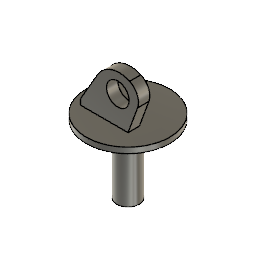
Assembly (Autodesk Fusion 360 archive; units mm, degrees)
design "Z rotation"
Autodesk Fusion 360 part; units mm, degrees
(part 1 of 5)
cylinder "CylinderPrimitive1" add diameter 20 height 60 placed x (1, 0, 0) y (0, 1, 0) z (0, 0, 1) at (0, 0, 0)
sketch "Sketch2" plane through (0, 0, 60) normal (0, 0, 1) x (-1, 0, 0)
  circle A0 centre (0, 0) radius 10
  circle A1 centre (0, 0) radius 37
  dimension "d3" = 74
  constraint coincident A0.centre A1.centre
  measures "d3" diameter of A1
extrude "Extrude1" add sketch "Sketch2" along normal blind 5 contours A0 | A1
sketch "Sketch3" plane through (0, 0, 0) normal (0, 1, 0) x (1, 0, 0)
  line L0 (-37, -65) -> (37, -65)
  line L1 (-27, -65) -> (-27, -70)
  line L2 (-27, -70) -> (-12, -95.9808)
  line L3 (-27, -70) -> (3, -70) construction
  line L4 (15.0513, -65) -> (23.4704, -88.1312)
  line L5 (-12, -95.9808) -> (26.3274, -95.9808) construction
  arc A0 (-12, -95.9808) -> (16.4497, -105.0022) centre (7.1637, -84.9166) ccw
  arc A1 (16.4497, -105.0022) -> (23.4704, -88.1312) centre (10.7845, -92.7484) ccw
  dimension "d6" = 5
  dimension "d8" = 30
  dimension "d9" = 10
  dimension "d12" = 74
  dimension "d15" = 60
  dimension "d16" = 70
  dimension "d17" = 13.5
  constraint coincident L0 L1.start
  constraint perpendicular L0 L1
  constraint horizontal L3
  constraint coincident L0 L4.start
  constraint horizontal L5
  constraint tangent L2 A0
  constraint coincident L4 L5.end
  constraint coincident L5.end A0
  constraint tangent L4 A1
  constraint tangent A0 A1
  measures "d6" distance of L1.start L1.end
  measures "d8" distance of L1.end L2.end
  measures "d9" distance of L0.start L1.start
  measures "d12" distance of L0.start L0.end
  measures "d15" angle of L2 L3
  measures "d16" angle of L0 L4
  measures "d17" radius of A1
extrude "Extrude2" add sketch "Sketch3" against normal blind 10 from surface at -5
hole "Hole1" at (6, -15, 90) direction (0, 1, 0) diameter 20 end through all

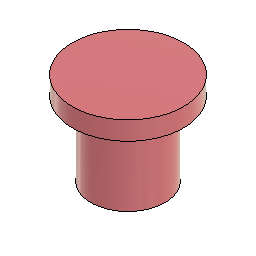
design "Pin"
Autodesk Fusion 360 part; units mm, degrees
sketch "Sketch1" plane through (0, 0, 0) normal (0, 0, 1) x (1, 0, 0)
  circle A0 centre (0, 0) radius 10
  dimension "d1" = 20
  constraint coincident A0.centre origin
  measures "d1" diameter of A0
extrude "Extrude1" add sketch "Sketch1" along normal blind 20
sketch "Sketch2" plane through (0, 0, 20) normal (0, 0, 1) x (-1, 0, 0)
  circle A0 centre (0, 0) radius 10
  circle A1 centre (0, 0) radius 15
  dimension "d4" = 30
  constraint coincident A0.centre A1.centre
  measures "d4" diameter of A1
extrude "Extrude2" add sketch "Sketch2" along normal blind 5 contours A0 | A1

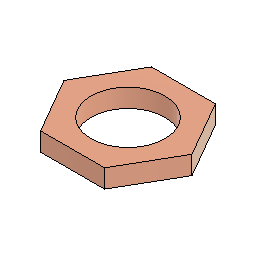
design "Hex"
Autodesk Fusion 360 part; units mm, degrees
sketch "Sketch1" plane through (0, 0, 0) normal (0, 0, 1) x (1, 0, 0)
  line L0 (8.6603, -15) -> (17.3205, 0)
  line L1 (17.3205, 0) -> (8.6603, 15)
  line L2 (8.6603, 15) -> (-8.6603, 15)
  line L3 (-8.6603, 15) -> (-17.3205, 0)
  line L4 (-17.3205, 0) -> (-8.6603, -15)
  line L5 (-8.6603, -15) -> (8.6603, -15)
  dimension "d1" = 15
  measures "d1" distance of origin L5
extrude "Extrude1" add sketch "Sketch1" along normal blind 5
hole "Hole1" at (0, 0, 5) direction (0, 0, -1) diameter 20 depth 20 tip angle 118

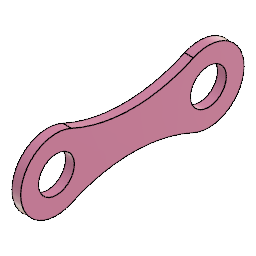
design "Yoke"
Autodesk Fusion 360 part; units mm, degrees
sketch "Sketch1" plane through (0, 0, 0) normal (1, 0, 0) x (0, 1, 0)
  circle A0 centre (0, 0) radius 20
  circle A1 centre (0, 0) radius 10
  line L0 (0, 0) -> (85, 0) construction
  circle A2 centre (85, 0) radius 20
  circle A3 centre (85, 0) radius 10
  arc A4 (8.3775, 18.1609) -> (76.6225, 18.1609) centre (42.5, 92.1318) ccw
  arc A5 (76.6225, -18.1609) -> (8.3775, -18.1609) centre (42.5, -92.1318) ccw
  dimension "d1" = 40
  dimension "d2" = 20
  dimension "d3" = 85
  dimension "d4" = 40
  dimension "d5" = 20
  constraint coincident A0.centre A1.centre
  constraint concentric A0 A1
  constraint horizontal L0
  constraint coincident L0.end A2.centre
  constraint concentric A2 A3
  constraint tangent A0 A4
  constraint tangent A2 A4
  constraint symmetric L0 A4 A5
  constraint coincident A2 A4.end
  constraint coincident A0 A4.start
  constraint coincident A0 A5.end
  constraint coincident A2 A5.start
  measures "d1" diameter of A0
  measures "d2" diameter of A1
  measures "d3" distance of A0.centre L0.end
  measures "d4" diameter of A2
  measures "d5" diameter of A3
extrude "Extrude1" add sketch "Sketch1" along normal blind 5

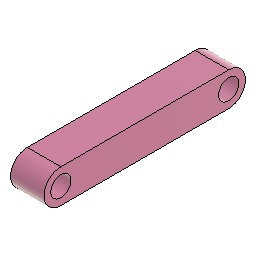
design "SmallYoke"
Autodesk Fusion 360 part; units mm, degrees
sketch "Sketch1" plane through (0, 0, 0) normal (1, 0, 0) x (0, 1, 0)
  circle A0 centre (0, 0) radius 2.5
  circle A1 centre (0, 0) radius 1.5
  line L0 (0, 0) -> (25, 0) construction
  circle A2 centre (25, 0) radius 2.5
  circle A3 centre (25, 0) radius 1.5
  line L1 (0, 2.5) -> (25, 2.5)
  line L2 (0, -2.5) -> (25, -2.5)
  dimension "d1" = 5
  dimension "d2" = 3
  dimension "d3" = 25
  dimension "d4" = 5
  dimension "d5" = 3
  constraint coincident A0.centre A1.centre
  constraint concentric A0 A1
  constraint horizontal L0
  constraint coincident L0.end A2.centre
  constraint concentric A2 A3
  constraint tangent A0 L1
  constraint tangent A2 L1
  constraint coincident A0 L1.start
  constraint coincident A2 L1.end
  constraint symmetric L0 L1.start L2.start
  constraint symmetric L0 L1.end L2.end
  measures "d1" diameter of A0
  measures "d2" diameter of A1
  measures "d3" distance of A0.centre L0.end
  measures "d4" diameter of A2
  measures "d5" diameter of A3
extrude "Extrude1" add sketch "Sketch1" along normal blind 5

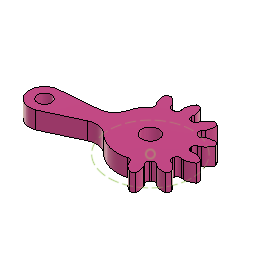
design "Spur Gear-Left"
description: Spur Gear; Module: 2.0; Num Teeth: 12; Pressure Angle: 20.0; Backlash: 0.00 mm
Autodesk Fusion 360 part; units mm, degrees
derive "DerivedContext1" from "Assembly v8"
sketch "Sketch1" plane through (0, 0, 0) normal (0, 0, 1) x (1, 0, 0) in component "Spur Gear (12 teeth)"
  circle A0 centre (0, 0) radius 9.5492
  circle A1 centre (0, 0) radius 2.5
extrude "Extrude1" add sketch "Sketch1" along normal blind 5 in component "Spur Gear (12 teeth)"
sketch "Sketch2" plane through (0, 0, 0) normal (0, 0, 1) x (1, 0, 0) in component "Spur Gear (12 teeth)"
  spline S0 degree 5 poles (11.1567, -1.6383) (11.1647, -1.6395) (11.1807, -1.6416) (11.2048, -1.6439) (11.237, -1.6456) (11.2774, -1.6458) (11.318, -1.6445) (11.3587, -1.6423) (11.3994, -1.6396) (11.4401, -1.6366) (11.4809, -1.6333) (11.5218, -1.6295) (11.5626, -1.625) (11.6035, -1.6199) (11.6445, -1.614) (11.6854, -1.6075) (11.7264, -1.6005) (11.7674, -1.5929) (11.8084, -1.585) (11.8494, -1.5766) (11.8905, -1.5678) (11.9315, -1.5587) (11.9725, -1.5491) (12.0135, -1.539) (12.0545, -1.5285) (12.0956, -1.5175) (12.1366, -1.5062) (12.1776, -1.4944) (12.2186, -1.4823) (12.2595, -1.4698) (12.3005, -1.4569) (12.3414, -1.4437) (12.3824, -1.4301) (12.4233, -1.4161) (12.4641, -1.4018) (12.505, -1.3871) (12.5458, -1.372) (12.5866, -1.3566) (12.6274, -1.3409) (12.6681, -1.3248) (12.7088, -1.3084) (12.7495, -1.2917) (12.7902, -1.2746) (12.8308, -1.2572) (12.8713, -1.2395) (12.9119, -1.2215) (12.9523, -1.2031) (12.9928, -1.1844) (13.0332, -1.1654) (13.0735, -1.1461) (13.1138, -1.1265) (13.1541, -1.1066) (13.1943, -1.0863) (13.2345, -1.0658) (13.2746, -1.045) (13.3146, -1.0239) (13.3546, -1.0024) (13.3946, -0.9807) (13.4344, -0.9587) (13.4743, -0.9364) (13.514, -0.9138) (13.5538, -0.8909) (13.5934, -0.8678) (13.633, -0.8443) (13.6725, -0.8206) (13.712, -0.7966) (13.7514, -0.7723) (13.7907, -0.7477) (13.8299, -0.7229) (13.8691, -0.6978) (13.9082, -0.6724) (13.9395, -0.6518) (13.9629, -0.6363) (13.9784, -0.6259) (13.9862, -0.6207) knots 0 0 0 0 0 0 0.01428571 0.02857143 0.04285714 0.05714286 0.07142857 0.08571429 0.1 0.11428571 0.12857143 0.14285714 0.15714286 0.17142857 0.18571429 0.2 0.21428571 0.22857143 0.24285714 0.25714286 0.27142857 0.28571429 0.3 0.31428571 0.32857143 0.34285714 0.35714286 0.37142857 0.38571429 0.4 0.41428571 0.42857143 0.44285714 0.45714286 0.47142857 0.48571429 0.5 0.51428571 0.52857143 0.54285714 0.55714286 0.57142857 0.58571429 0.6 0.61428571 0.62857143 0.64285714 0.65714286 0.67142857 0.68571429 0.7 0.71428571 0.72857143 0.74285714 0.75714286 0.77142857 0.78571429 0.8 0.81428571 0.82857143 0.84285714 0.85714286 0.87142857 0.88571429 0.9 0.91428571 0.92857143 0.94285714 0.95714286 0.97142857 0.98571429 1 1 1 1 1 1
  spline S1 degree 5 poles (11.1567, 1.6383) (11.1647, 1.6395) (11.1807, 1.6416) (11.2048, 1.6439) (11.237, 1.6456) (11.2774, 1.6458) (11.318, 1.6445) (11.3587, 1.6423) (11.3994, 1.6396) (11.4401, 1.6366) (11.4809, 1.6333) (11.5218, 1.6295) (11.5626, 1.625) (11.6035, 1.6199) (11.6445, 1.614) (11.6854, 1.6075) (11.7264, 1.6005) (11.7674, 1.5929) (11.8084, 1.585) (11.8494, 1.5766) (11.8905, 1.5678) (11.9315, 1.5587) (11.9725, 1.5491) (12.0135, 1.539) (12.0545, 1.5285) (12.0956, 1.5175) (12.1366, 1.5062) (12.1776, 1.4944) (12.2186, 1.4823) (12.2595, 1.4698) (12.3005, 1.4569) (12.3414, 1.4437) (12.3824, 1.4301) (12.4233, 1.4161) (12.4641, 1.4018) (12.505, 1.3871) (12.5458, 1.372) (12.5866, 1.3566) (12.6274, 1.3409) (12.6681, 1.3248) (12.7088, 1.3084) (12.7495, 1.2917) (12.7902, 1.2746) (12.8308, 1.2572) (12.8713, 1.2395) (12.9119, 1.2215) (12.9523, 1.2031) (12.9928, 1.1844) (13.0332, 1.1654) (13.0735, 1.1461) (13.1138, 1.1265) (13.1541, 1.1066) (13.1943, 1.0863) (13.2345, 1.0658) (13.2746, 1.045) (13.3146, 1.0239) (13.3546, 1.0024) (13.3946, 0.9807) (13.4344, 0.9587) (13.4743, 0.9364) (13.514, 0.9138) (13.5538, 0.8909) (13.5934, 0.8678) (13.633, 0.8443) (13.6725, 0.8206) (13.712, 0.7966) (13.7514, 0.7723) (13.7907, 0.7477) (13.8299, 0.7229) (13.8691, 0.6978) (13.9082, 0.6724) (13.9395, 0.6518) (13.9629, 0.6363) (13.9784, 0.6259) (13.9862, 0.6207) knots 0 0 0 0 0 0 0.01428571 0.02857143 0.04285714 0.05714286 0.07142857 0.08571429 0.1 0.11428571 0.12857143 0.14285714 0.15714286 0.17142857 0.18571429 0.2 0.21428571 0.22857143 0.24285714 0.25714286 0.27142857 0.28571429 0.3 0.31428571 0.32857143 0.34285714 0.35714286 0.37142857 0.38571429 0.4 0.41428571 0.42857143 0.44285714 0.45714286 0.47142857 0.48571429 0.5 0.51428571 0.52857143 0.54285714 0.55714286 0.57142857 0.58571429 0.6 0.61428571 0.62857143 0.64285714 0.65714286 0.67142857 0.68571429 0.7 0.71428571 0.72857143 0.74285714 0.75714286 0.77142857 0.78571429 0.8 0.81428571 0.82857143 0.84285714 0.85714286 0.87142857 0.88571429 0.9 0.91428571 0.92857143 0.94285714 0.95714286 0.97142857 0.98571429 1 1 1 1 1 1
  arc A0 (13.9862, -0.6207) -> (13.9862, 0.6207) centre (0, 0) ccw
  line L0 (9.438, -1.3874) -> (11.1567, -1.6383)
  line L1 (9.438, 1.3874) -> (11.1567, 1.6383)
  line L2 (9.438, -1.3874) -> (9.438, 1.3874)
  point P0 (11.3527, -1.6425)
  point P1 (11.5515, -1.6261)
  point P2 (11.7521, -1.5957)
  point P3 (11.954, -1.5533)
  point P4 (12.1568, -1.5003)
  point P5 (12.3603, -1.4374)
  point P6 (12.5642, -1.3651)
  point P7 (12.7683, -1.2838)
  point P8 (12.9724, -1.1938)
  point P9 (13.1764, -1.0953)
  point P10 (13.3799, -0.9887)
  point P11 (13.5828, -0.8739)
  point P12 (13.785, -0.7512)
  point P13 (11.3527, 1.6425)
  point P14 (11.5515, 1.6261)
  point P15 (11.7521, 1.5957)
  point P16 (11.954, 1.5533)
  point P17 (12.1568, 1.5003)
  point P18 (12.3603, 1.4374)
  point P19 (12.5642, 1.3651)
  point P20 (12.7683, 1.2838)
  point P21 (12.9724, 1.1938)
  point P22 (13.1764, 1.0953)
  point P23 (13.3799, 0.9887)
  point P24 (13.5828, 0.8739)
  point P25 (13.785, 0.7512)
extrude "Extrude2" add sketch "Sketch2" along normal blind 5 in component "Spur Gear (12 teeth)"
fillet "Fillet1" radius 1 2 edges at (9.4477, -1.3888, 2.5) (9.4477, 1.3888, 2.5) in component "Spur Gear (12 teeth)"
pattern_circular "C-Pattern1" count 12 over 360 about axis through (0, 0, 0) along (0, 0, 1) of "Extrude2", "Fillet1" in component "Spur Gear (12 teeth)"
sketch "Sketch3" plane through (0, 0, 0) normal (0, 0, 1) x (1, 0, 0) in component "Spur Gear (12 teeth)"
  circle A0 centre (0, 0) radius 12 construction
sketch "Sketch1 (2)" plane through (0, 0, 5) normal (0, 0, 1) x (-1, 0, 0)
  arc A0 (-9.1699, 2.6646) -> (-9.2737, 2.2773) centre (0, 0) ccw
  arc A1 (-10.3893, 1.5263) -> (-9.2737, 2.2773) centre (-10.2448, 2.5158) ccw
  line L0 (-10.3893, 1.5263) -> (-11.1567, 1.6383)
  spline S0 degree 5 poles (-11.1567, 1.6383) (-11.1647, 1.6395) (-11.1807, 1.6416) (-11.2048, 1.6439) (-11.237, 1.6456) (-11.2774, 1.6458) (-11.318, 1.6445) (-11.3587, 1.6423) (-11.3994, 1.6396) (-11.4401, 1.6366) (-11.4809, 1.6333) (-11.5218, 1.6295) (-11.5626, 1.625) (-11.6035, 1.6199) (-11.6445, 1.614) (-11.6854, 1.6075) (-11.7264, 1.6005) (-11.7674, 1.5929) (-11.8084, 1.585) (-11.8494, 1.5766) (-11.8905, 1.5678) (-11.9315, 1.5587) (-11.9725, 1.5491) (-12.0135, 1.539) (-12.0545, 1.5285) (-12.0956, 1.5175) (-12.1366, 1.5062) (-12.1776, 1.4944) (-12.2186, 1.4823) (-12.2595, 1.4698) (-12.3005, 1.4569) (-12.3414, 1.4437) (-12.3824, 1.4301) (-12.4233, 1.4161) (-12.4641, 1.4018) (-12.505, 1.3871) (-12.5458, 1.372) (-12.5866, 1.3566) (-12.6274, 1.3409) (-12.6681, 1.3248) (-12.7088, 1.3084) (-12.7495, 1.2917) (-12.7902, 1.2746) (-12.8308, 1.2572) (-12.8713, 1.2395) (-12.9119, 1.2215) (-12.9523, 1.2031) (-12.9928, 1.1844) (-13.0332, 1.1654) (-13.0735, 1.1461) (-13.1138, 1.1265) (-13.1541, 1.1066) (-13.1943, 1.0863) (-13.2345, 1.0658) (-13.2746, 1.045) (-13.3146, 1.0239) (-13.3546, 1.0024) (-13.3946, 0.9807) (-13.4344, 0.9587) (-13.4743, 0.9364) (-13.514, 0.9138) (-13.5538, 0.8909) (-13.5934, 0.8678) (-13.633, 0.8443) (-13.6725, 0.8206) (-13.712, 0.7966) (-13.7514, 0.7723) (-13.7907, 0.7477) (-13.8299, 0.7229) (-13.8691, 0.6978) (-13.9082, 0.6724) (-13.9395, 0.6518) (-13.9629, 0.6363) (-13.9784, 0.6259) (-13.9862, 0.6207) knots 0 0 0 0 0 0 0.01428571 0.02857143 0.04285714 0.05714286 0.07142857 0.08571429 0.1 0.11428571 0.12857143 0.14285714 0.15714286 0.17142857 0.18571429 0.2 0.21428571 0.22857143 0.24285714 0.25714286 0.27142857 0.28571429 0.3 0.31428571 0.32857143 0.34285714 0.35714286 0.37142857 0.38571429 0.4 0.41428571 0.42857143 0.44285714 0.45714286 0.47142857 0.48571429 0.5 0.51428571 0.52857143 0.54285714 0.55714286 0.57142857 0.58571429 0.6 0.61428571 0.62857143 0.64285714 0.65714286 0.67142857 0.68571429 0.7 0.71428571 0.72857143 0.74285714 0.75714286 0.77142857 0.78571429 0.8 0.81428571 0.82857143 0.84285714 0.85714286 0.87142857 0.88571429 0.9 0.91428571 0.92857143 0.94285714 0.95714286 0.97142857 0.98571429 1 1 1 1 1 1
  arc A2 (-13.9862, 0.6207) -> (-13.9862, -0.6207) centre (0, 0) ccw
  spline S1 degree 5 poles (-13.9862, -0.6207) (-13.9784, -0.6259) (-13.9629, -0.6363) (-13.9395, -0.6518) (-13.9082, -0.6724) (-13.8691, -0.6978) (-13.8299, -0.7229) (-13.7907, -0.7477) (-13.7514, -0.7723) (-13.712, -0.7966) (-13.6725, -0.8206) (-13.633, -0.8443) (-13.5934, -0.8678) (-13.5538, -0.8909) (-13.514, -0.9138) (-13.4743, -0.9364) (-13.4344, -0.9587) (-13.3946, -0.9807) (-13.3546, -1.0024) (-13.3146, -1.0239) (-13.2746, -1.045) (-13.2345, -1.0658) (-13.1943, -1.0863) (-13.1541, -1.1066) (-13.1138, -1.1265) (-13.0735, -1.1461) (-13.0332, -1.1654) (-12.9928, -1.1844) (-12.9523, -1.2031) (-12.9119, -1.2215) (-12.8713, -1.2395) (-12.8308, -1.2572) (-12.7902, -1.2746) (-12.7495, -1.2917) (-12.7088, -1.3084) (-12.6681, -1.3248) (-12.6274, -1.3409) (-12.5866, -1.3566) (-12.5458, -1.372) (-12.505, -1.3871) (-12.4641, -1.4018) (-12.4233, -1.4161) (-12.3824, -1.4301) (-12.3414, -1.4437) (-12.3005, -1.4569) (-12.2595, -1.4698) (-12.2186, -1.4823) (-12.1776, -1.4944) (-12.1366, -1.5062) (-12.0956, -1.5175) (-12.0545, -1.5285) (-12.0135, -1.539) (-11.9725, -1.5491) (-11.9315, -1.5587) (-11.8905, -1.5678) (-11.8494, -1.5766) (-11.8084, -1.585) (-11.7674, -1.5929) (-11.7264, -1.6005) (-11.6854, -1.6075) (-11.6445, -1.614) (-11.6035, -1.6199) (-11.5626, -1.625) (-11.5218, -1.6295) (-11.4809, -1.6333) (-11.4401, -1.6366) (-11.3994, -1.6396) (-11.3587, -1.6423) (-11.318, -1.6445) (-11.2774, -1.6458) (-11.237, -1.6456) (-11.2048, -1.6439) (-11.1807, -1.6416) (-11.1647, -1.6395) (-11.1567, -1.6383) knots -1 -1 -1 -1 -1 -1 -0.98571429 -0.97142857 -0.95714286 -0.94285714 -0.92857143 -0.91428571 -0.9 -0.88571429 -0.87142857 -0.85714286 -0.84285714 -0.82857143 -0.81428571 -0.8 -0.78571429 -0.77142857 -0.75714286 -0.74285714 -0.72857143 -0.71428571 -0.7 -0.68571429 -0.67142857 -0.65714286 -0.64285714 -0.62857143 -0.61428571 -0.6 -0.58571429 -0.57142857 -0.55714286 -0.54285714 -0.52857143 -0.51428571 -0.5 -0.48571429 -0.47142857 -0.45714286 -0.44285714 -0.42857143 -0.41428571 -0.4 -0.38571429 -0.37142857 -0.35714286 -0.34285714 -0.32857143 -0.31428571 -0.3 -0.28571429 -0.27142857 -0.25714286 -0.24285714 -0.22857143 -0.21428571 -0.2 -0.18571429 -0.17142857 -0.15714286 -0.14285714 -0.12857143 -0.11428571 -0.1 -0.08571429 -0.07142857 -0.05714286 -0.04285714 -0.02857143 -0.01428571 0 0 0 0 0 0
  line L1 (-11.1567, -1.6383) -> (-10.3893, -1.5263)
  arc A3 (-9.2737, -2.2773) -> (-10.3893, -1.5263) centre (-10.2448, -2.5158) ccw
  arc A4 (-9.2737, -2.2773) -> (-9.1699, -2.6646) centre (0, 0) ccw
  arc A5 (-9.7605, -3.8729) -> (-9.1699, -2.6646) centre (-10.1302, -2.9437) ccw
  line L2 (-9.7605, -3.8729) -> (-10.4811, -4.1595)
  spline S2 degree 5 poles (-10.4811, -4.1595) (-10.4886, -4.1625) (-10.5035, -4.1687) (-10.5256, -4.1787) (-10.5543, -4.1933) (-10.5894, -4.2134) (-10.6239, -4.2349) (-10.658, -4.2571) (-10.692, -4.2797) (-10.7258, -4.3027) (-10.7594, -4.326) (-10.7929, -4.3497) (-10.826, -4.374) (-10.8589, -4.3989) (-10.8914, -4.4244) (-10.9236, -4.4505) (-10.9556, -4.4772) (-10.9873, -4.5042) (-11.0189, -4.5316) (-11.0502, -4.5593) (-11.0814, -4.5874) (-11.1123, -4.6159) (-11.143, -4.6447) (-11.1735, -4.674) (-11.2038, -4.7036) (-11.2338, -4.7336) (-11.2637, -4.7639) (-11.2933, -4.7946) (-11.3227, -4.8256) (-11.352, -4.8569) (-11.381, -4.8885) (-11.4099, -4.9204) (-11.4385, -4.9527) (-11.4669, -4.9852) (-11.4952, -5.0181) (-11.5232, -5.0512) (-11.551, -5.0847) (-11.5787, -5.1184) (-11.6061, -5.1524) (-11.6334, -5.1867) (-11.6604, -5.2213) (-11.6873, -5.2561) (-11.7139, -5.2912) (-11.7404, -5.3266) (-11.7666, -5.3622) (-11.7927, -5.3981) (-11.8186, -5.4343) (-11.8443, -5.4707) (-11.8698, -5.5073) (-11.8951, -5.5442) (-11.9202, -5.5813) (-11.9451, -5.6187) (-11.9698, -5.6563) (-11.9943, -5.6942) (-12.0186, -5.7323) (-12.0427, -5.7706) (-12.0667, -5.8092) (-12.0904, -5.848) (-12.1139, -5.887) (-12.1373, -5.9262) (-12.1604, -5.9656) (-12.1834, -6.0053) (-12.2061, -6.0452) (-12.2287, -6.0853) (-12.251, -6.1256) (-12.2732, -6.1661) (-12.2952, -6.2069) (-12.3169, -6.2478) (-12.3385, -6.2889) (-12.3599, -6.3303) (-12.3811, -6.3718) (-12.3979, -6.4052) (-12.4104, -6.4304) (-12.4186, -6.4472) (-12.4228, -6.4556) knots 0 0 0 0 0 0 0.01428571 0.02857143 0.04285714 0.05714286 0.07142857 0.08571429 0.1 0.11428571 0.12857143 0.14285714 0.15714286 0.17142857 0.18571429 0.2 0.21428571 0.22857143 0.24285714 0.25714286 0.27142857 0.28571429 0.3 0.31428571 0.32857143 0.34285714 0.35714286 0.37142857 0.38571429 0.4 0.41428571 0.42857143 0.44285714 0.45714286 0.47142857 0.48571429 0.5 0.51428571 0.52857143 0.54285714 0.55714286 0.57142857 0.58571429 0.6 0.61428571 0.62857143 0.64285714 0.65714286 0.67142857 0.68571429 0.7 0.71428571 0.72857143 0.74285714 0.75714286 0.77142857 0.78571429 0.8 0.81428571 0.82857143 0.84285714 0.85714286 0.87142857 0.88571429 0.9 0.91428571 0.92857143 0.94285714 0.95714286 0.97142857 0.98571429 1 1 1 1 1 1
  arc A6 (-12.4228, -6.4556) -> (-11.8021, -7.5307) centre (0, 0) ccw
  spline S3 degree 5 poles (-11.8021, -7.5307) (-11.7927, -7.5313) (-11.774, -7.5325) (-11.746, -7.5342) (-11.7087, -7.5364) (-11.6621, -7.5388) (-11.6156, -7.541) (-11.5692, -7.5429) (-11.5229, -7.5445) (-11.4766, -7.5458) (-11.4305, -7.5469) (-11.3844, -7.5477) (-11.3384, -7.5482) (-11.2924, -7.5484) (-11.2466, -7.5484) (-11.2009, -7.5481) (-11.1552, -7.5475) (-11.1097, -7.5466) (-11.0642, -7.5454) (-11.0189, -7.544) (-10.9736, -7.5423) (-10.9285, -7.5403) (-10.8834, -7.538) (-10.8385, -7.5354) (-10.7937, -7.5325) (-10.7489, -7.5293) (-10.7044, -7.5259) (-10.6599, -7.5221) (-10.6155, -7.5181) (-10.5713, -7.5137) (-10.5271, -7.5091) (-10.4832, -7.5042) (-10.4393, -7.4989) (-10.3956, -7.4934) (-10.352, -7.4876) (-10.3085, -7.4814) (-10.2652, -7.475) (-10.222, -7.4682) (-10.179, -7.4611) (-10.1361, -7.4538) (-10.0934, -7.4461) (-10.0508, -7.438) (-10.0084, -7.4297) (-9.9662, -7.421) (-9.9241, -7.412) (-9.8822, -7.4027) (-9.8404, -7.393) (-9.7989, -7.383) (-9.7575, -7.3727) (-9.7163, -7.362) (-9.6753, -7.351) (-9.6345, -7.3396) (-9.594, -7.3278) (-9.5536, -7.3156) (-9.5135, -7.303) (-9.4736, -7.2901) (-9.4339, -7.2768) (-9.3944, -7.2632) (-9.3551, -7.2492) (-9.3161, -7.2349) (-9.2774, -7.22) (-9.239, -7.2046) (-9.201, -7.1886) (-9.1634, -7.172) (-9.1261, -7.1549) (-9.0891, -7.1374) (-9.0523, -7.1196) (-9.0157, -7.1016) (-8.9794, -7.0831) (-8.9437, -7.064) (-8.9087, -7.0436) (-8.8816, -7.0261) (-8.862, -7.012) (-8.8491, -7.0022) (-8.8428, -6.9972) knots -1 -1 -1 -1 -1 -1 -0.98571429 -0.97142857 -0.95714286 -0.94285714 -0.92857143 -0.91428571 -0.9 -0.88571429 -0.87142857 -0.85714286 -0.84285714 -0.82857143 -0.81428571 -0.8 -0.78571429 -0.77142857 -0.75714286 -0.74285714 -0.72857143 -0.71428571 -0.7 -0.68571429 -0.67142857 -0.65714286 -0.64285714 -0.62857143 -0.61428571 -0.6 -0.58571429 -0.57142857 -0.55714286 -0.54285714 -0.52857143 -0.51428571 -0.5 -0.48571429 -0.47142857 -0.45714286 -0.44285714 -0.42857143 -0.41428571 -0.4 -0.38571429 -0.37142857 -0.35714286 -0.34285714 -0.32857143 -0.31428571 -0.3 -0.28571429 -0.27142857 -0.25714286 -0.24285714 -0.22857143 -0.21428571 -0.2 -0.18571429 -0.17142857 -0.15714286 -0.14285714 -0.12857143 -0.11428571 -0.1 -0.08571429 -0.07142857 -0.05714286 -0.04285714 -0.02857143 -0.01428571 0 0 0 0 0 0
  line L3 (-8.8428, -6.9972) -> (-8.2343, -6.5164)
  arc A7 (-6.8926, -6.609) -> (-8.2343, -6.5164) centre (-7.6144, -7.3011) ccw
  arc A8 (-6.8926, -6.609) -> (-6.609, -6.8926) centre (0, 0) ccw
  arc A9 (-6.5164, -8.2343) -> (-6.609, -6.8926) centre (-7.3011, -7.6144) ccw
  line L4 (-6.5164, -8.2343) -> (-6.9972, -8.8428)
  spline S4 degree 5 poles (-6.9972, -8.8428) (-7.0022, -8.8491) (-7.012, -8.862) (-7.0261, -8.8816) (-7.0436, -8.9087) (-7.064, -8.9437) (-7.0831, -8.9794) (-7.1016, -9.0157) (-7.1196, -9.0523) (-7.1374, -9.0891) (-7.1549, -9.1261) (-7.172, -9.1634) (-7.1886, -9.201) (-7.2046, -9.239) (-7.22, -9.2774) (-7.2349, -9.3161) (-7.2492, -9.3551) (-7.2632, -9.3944) (-7.2768, -9.4339) (-7.2901, -9.4736) (-7.303, -9.5135) (-7.3156, -9.5536) (-7.3278, -9.594) (-7.3396, -9.6345) (-7.351, -9.6753) (-7.362, -9.7163) (-7.3727, -9.7575) (-7.383, -9.7989) (-7.393, -9.8404) (-7.4027, -9.8822) (-7.412, -9.9241) (-7.421, -9.9662) (-7.4297, -10.0084) (-7.438, -10.0508) (-7.4461, -10.0934) (-7.4538, -10.1361) (-7.4611, -10.179) (-7.4682, -10.222) (-7.475, -10.2652) (-7.4814, -10.3085) (-7.4876, -10.352) (-7.4934, -10.3956) (-7.4989, -10.4393) (-7.5042, -10.4832) (-7.5091, -10.5271) (-7.5137, -10.5713) (-7.5181, -10.6155) (-7.5221, -10.6599) (-7.5259, -10.7044) (-7.5293, -10.7489) (-7.5325, -10.7937) (-7.5354, -10.8385) (-7.538, -10.8834) (-7.5403, -10.9285) (-7.5423, -10.9736) (-7.544, -11.0189) (-7.5454, -11.0642) (-7.5466, -11.1097) (-7.5475, -11.1552) (-7.5481, -11.2009) (-7.5484, -11.2466) (-7.5484, -11.2924) (-7.5482, -11.3384) (-7.5477, -11.3844) (-7.5469, -11.4305) (-7.5458, -11.4766) (-7.5445, -11.5229) (-7.5429, -11.5692) (-7.541, -11.6156) (-7.5388, -11.6621) (-7.5364, -11.7087) (-7.5342, -11.746) (-7.5325, -11.774) (-7.5313, -11.7927) (-7.5307, -11.8021) knots 0 0 0 0 0 0 0.01428571 0.02857143 0.04285714 0.05714286 0.07142857 0.08571429 0.1 0.11428571 0.12857143 0.14285714 0.15714286 0.17142857 0.18571429 0.2 0.21428571 0.22857143 0.24285714 0.25714286 0.27142857 0.28571429 0.3 0.31428571 0.32857143 0.34285714 0.35714286 0.37142857 0.38571429 0.4 0.41428571 0.42857143 0.44285714 0.45714286 0.47142857 0.48571429 0.5 0.51428571 0.52857143 0.54285714 0.55714286 0.57142857 0.58571429 0.6 0.61428571 0.62857143 0.64285714 0.65714286 0.67142857 0.68571429 0.7 0.71428571 0.72857143 0.74285714 0.75714286 0.77142857 0.78571429 0.8 0.81428571 0.82857143 0.84285714 0.85714286 0.87142857 0.88571429 0.9 0.91428571 0.92857143 0.94285714 0.95714286 0.97142857 0.98571429 1 1 1 1 1 1
  arc A10 (-7.5307, -11.8021) -> (-6.4556, -12.4228) centre (0, 0) ccw
  spline S5 degree 5 poles (-6.4556, -12.4228) (-6.4472, -12.4186) (-6.4304, -12.4104) (-6.4052, -12.3979) (-6.3718, -12.3811) (-6.3303, -12.3599) (-6.2889, -12.3385) (-6.2478, -12.3169) (-6.2069, -12.2952) (-6.1661, -12.2732) (-6.1256, -12.251) (-6.0853, -12.2287) (-6.0452, -12.2061) (-6.0053, -12.1834) (-5.9656, -12.1604) (-5.9262, -12.1373) (-5.887, -12.1139) (-5.848, -12.0904) (-5.8092, -12.0667) (-5.7706, -12.0427) (-5.7323, -12.0186) (-5.6942, -11.9943) (-5.6563, -11.9698) (-5.6187, -11.9451) (-5.5813, -11.9202) (-5.5442, -11.8951) (-5.5073, -11.8698) (-5.4707, -11.8443) (-5.4343, -11.8186) (-5.3981, -11.7927) (-5.3622, -11.7666) (-5.3266, -11.7404) (-5.2912, -11.7139) (-5.2561, -11.6873) (-5.2213, -11.6604) (-5.1867, -11.6334) (-5.1524, -11.6061) (-5.1184, -11.5787) (-5.0847, -11.551) (-5.0512, -11.5232) (-5.0181, -11.4952) (-4.9852, -11.4669) (-4.9527, -11.4385) (-4.9204, -11.4099) (-4.8885, -11.381) (-4.8569, -11.352) (-4.8256, -11.3227) (-4.7946, -11.2933) (-4.7639, -11.2637) (-4.7336, -11.2338) (-4.7036, -11.2038) (-4.674, -11.1735) (-4.6447, -11.143) (-4.6159, -11.1123) (-4.5874, -11.0814) (-4.5593, -11.0502) (-4.5316, -11.0189) (-4.5042, -10.9873) (-4.4772, -10.9556) (-4.4505, -10.9236) (-4.4244, -10.8914) (-4.3989, -10.8589) (-4.374, -10.826) (-4.3497, -10.7929) (-4.326, -10.7594) (-4.3027, -10.7258) (-4.2797, -10.692) (-4.2571, -10.658) (-4.2349, -10.6239) (-4.2134, -10.5894) (-4.1933, -10.5543) (-4.1787, -10.5256) (-4.1687, -10.5035) (-4.1625, -10.4886) (-4.1595, -10.4811) knots -1 -1 -1 -1 -1 -1 -0.98571429 -0.97142857 -0.95714286 -0.94285714 -0.92857143 -0.91428571 -0.9 -0.88571429 -0.87142857 -0.85714286 -0.84285714 -0.82857143 -0.81428571 -0.8 -0.78571429 -0.77142857 -0.75714286 -0.74285714 -0.72857143 -0.71428571 -0.7 -0.68571429 -0.67142857 -0.65714286 -0.64285714 -0.62857143 -0.61428571 -0.6 -0.58571429 -0.57142857 -0.55714286 -0.54285714 -0.52857143 -0.51428571 -0.5 -0.48571429 -0.47142857 -0.45714286 -0.44285714 -0.42857143 -0.41428571 -0.4 -0.38571429 -0.37142857 -0.35714286 -0.34285714 -0.32857143 -0.31428571 -0.3 -0.28571429 -0.27142857 -0.25714286 -0.24285714 -0.22857143 -0.21428571 -0.2 -0.18571429 -0.17142857 -0.15714286 -0.14285714 -0.12857143 -0.11428571 -0.1 -0.08571429 -0.07142857 -0.05714286 -0.04285714 -0.02857143 -0.01428571 0 0 0 0 0 0
  line L5 (-4.1595, -10.4811) -> (-3.8729, -9.7605)
  arc A11 (-2.6646, -9.1699) -> (-3.8729, -9.7605) centre (-2.9437, -10.1302) ccw
  arc A12 (-2.6646, -9.1699) -> (-2.2773, -9.2737) centre (0, 0) ccw
  arc A13 (-1.5263, -10.3893) -> (-2.2773, -9.2737) centre (-2.5158, -10.2448) ccw
  line L6 (-1.5263, -10.3893) -> (-1.6383, -11.1567)
  spline S6 degree 5 poles (-1.6383, -11.1567) (-1.6395, -11.1647) (-1.6416, -11.1807) (-1.6439, -11.2048) (-1.6456, -11.237) (-1.6458, -11.2774) (-1.6445, -11.318) (-1.6423, -11.3587) (-1.6396, -11.3994) (-1.6366, -11.4401) (-1.6333, -11.4809) (-1.6295, -11.5218) (-1.625, -11.5626) (-1.6199, -11.6035) (-1.614, -11.6445) (-1.6075, -11.6854) (-1.6005, -11.7264) (-1.5929, -11.7674) (-1.585, -11.8084) (-1.5766, -11.8494) (-1.5678, -11.8905) (-1.5587, -11.9315) (-1.5491, -11.9725) (-1.539, -12.0135) (-1.5285, -12.0545) (-1.5175, -12.0956) (-1.5062, -12.1366) (-1.4944, -12.1776) (-1.4823, -12.2186) (-1.4698, -12.2595) (-1.4569, -12.3005) (-1.4437, -12.3414) (-1.4301, -12.3824) (-1.4161, -12.4233) (-1.4018, -12.4641) (-1.3871, -12.505) (-1.372, -12.5458) (-1.3566, -12.5866) (-1.3409, -12.6274) (-1.3248, -12.6681) (-1.3084, -12.7088) (-1.2917, -12.7495) (-1.2746, -12.7902) (-1.2572, -12.8308) (-1.2395, -12.8713) (-1.2215, -12.9119) (-1.2031, -12.9523) (-1.1844, -12.9928) (-1.1654, -13.0332) (-1.1461, -13.0735) (-1.1265, -13.1138) (-1.1066, -13.1541) (-1.0863, -13.1943) (-1.0658, -13.2345) (-1.045, -13.2746) (-1.0239, -13.3146) (-1.0024, -13.3546) (-0.9807, -13.3946) (-0.9587, -13.4344) (-0.9364, -13.4743) (-0.9138, -13.514) (-0.8909, -13.5538) (-0.8678, -13.5934) (-0.8443, -13.633) (-0.8206, -13.6725) (-0.7966, -13.712) (-0.7723, -13.7514) (-0.7477, -13.7907) (-0.7229, -13.8299) (-0.6978, -13.8691) (-0.6724, -13.9082) (-0.6518, -13.9395) (-0.6363, -13.9629) (-0.6259, -13.9784) (-0.6207, -13.9862) knots 0 0 0 0 0 0 0.01428571 0.02857143 0.04285714 0.05714286 0.07142857 0.08571429 0.1 0.11428571 0.12857143 0.14285714 0.15714286 0.17142857 0.18571429 0.2 0.21428571 0.22857143 0.24285714 0.25714286 0.27142857 0.28571429 0.3 0.31428571 0.32857143 0.34285714 0.35714286 0.37142857 0.38571429 0.4 0.41428571 0.42857143 0.44285714 0.45714286 0.47142857 0.48571429 0.5 0.51428571 0.52857143 0.54285714 0.55714286 0.57142857 0.58571429 0.6 0.61428571 0.62857143 0.64285714 0.65714286 0.67142857 0.68571429 0.7 0.71428571 0.72857143 0.74285714 0.75714286 0.77142857 0.78571429 0.8 0.81428571 0.82857143 0.84285714 0.85714286 0.87142857 0.88571429 0.9 0.91428571 0.92857143 0.94285714 0.95714286 0.97142857 0.98571429 1 1 1 1 1 1
  arc A14 (-0.6207, -13.9862) -> (0.6207, -13.9862) centre (0, 0) ccw
  spline S7 degree 5 poles (0.6207, -13.9862) (0.6259, -13.9784) (0.6363, -13.9629) (0.6518, -13.9395) (0.6724, -13.9082) (0.6978, -13.8691) (0.7229, -13.8299) (0.7477, -13.7907) (0.7723, -13.7514) (0.7966, -13.712) (0.8206, -13.6725) (0.8443, -13.633) (0.8678, -13.5934) (0.8909, -13.5538) (0.9138, -13.514) (0.9364, -13.4743) (0.9587, -13.4344) (0.9807, -13.3946) (1.0024, -13.3546) (1.0239, -13.3146) (1.045, -13.2746) (1.0658, -13.2345) (1.0863, -13.1943) (1.1066, -13.1541) (1.1265, -13.1138) (1.1461, -13.0735) (1.1654, -13.0332) (1.1844, -12.9928) (1.2031, -12.9523) (1.2215, -12.9119) (1.2395, -12.8713) (1.2572, -12.8308) (1.2746, -12.7902) (1.2917, -12.7495) (1.3084, -12.7088) (1.3248, -12.6681) (1.3409, -12.6274) (1.3566, -12.5866) (1.372, -12.5458) (1.3871, -12.505) (1.4018, -12.4641) (1.4161, -12.4233) (1.4301, -12.3824) (1.4437, -12.3414) (1.4569, -12.3005) (1.4698, -12.2595) (1.4823, -12.2186) (1.4944, -12.1776) (1.5062, -12.1366) (1.5175, -12.0956) (1.5285, -12.0545) (1.539, -12.0135) (1.5491, -11.9725) (1.5587, -11.9315) (1.5678, -11.8905) (1.5766, -11.8494) (1.585, -11.8084) (1.5929, -11.7674) (1.6005, -11.7264) (1.6075, -11.6854) (1.614, -11.6445) (1.6199, -11.6035) (1.625, -11.5626) (1.6295, -11.5218) (1.6333, -11.4809) (1.6366, -11.4401) (1.6396, -11.3994) (1.6423, -11.3587) (1.6445, -11.318) (1.6458, -11.2774) (1.6456, -11.237) (1.6439, -11.2048) (1.6416, -11.1807) (1.6395, -11.1647) (1.6383, -11.1567) knots -1 -1 -1 -1 -1 -1 -0.98571429 -0.97142857 -0.95714286 -0.94285714 -0.92857143 -0.91428571 -0.9 -0.88571429 -0.87142857 -0.85714286 -0.84285714 -0.82857143 -0.81428571 -0.8 -0.78571429 -0.77142857 -0.75714286 -0.74285714 -0.72857143 -0.71428571 -0.7 -0.68571429 -0.67142857 -0.65714286 -0.64285714 -0.62857143 -0.61428571 -0.6 -0.58571429 -0.57142857 -0.55714286 -0.54285714 -0.52857143 -0.51428571 -0.5 -0.48571429 -0.47142857 -0.45714286 -0.44285714 -0.42857143 -0.41428571 -0.4 -0.38571429 -0.37142857 -0.35714286 -0.34285714 -0.32857143 -0.31428571 -0.3 -0.28571429 -0.27142857 -0.25714286 -0.24285714 -0.22857143 -0.21428571 -0.2 -0.18571429 -0.17142857 -0.15714286 -0.14285714 -0.12857143 -0.11428571 -0.1 -0.08571429 -0.07142857 -0.05714286 -0.04285714 -0.02857143 -0.01428571 0 0 0 0 0 0
  line L7 (1.6383, -11.1567) -> (1.5263, -10.3893)
  arc A15 (2.2773, -9.2737) -> (1.5263, -10.3893) centre (2.5158, -10.2448) ccw
  arc A16 (2.2773, -9.2737) -> (2.6646, -9.1699) centre (0, 0) ccw
  arc A17 (3.8729, -9.7605) -> (2.6646, -9.1699) centre (2.9437, -10.1302) ccw
  line L8 (3.8729, -9.7605) -> (4.1595, -10.4811)
  spline S8 degree 5 poles (4.1595, -10.4811) (4.1625, -10.4886) (4.1687, -10.5035) (4.1787, -10.5256) (4.1933, -10.5543) (4.2134, -10.5894) (4.2349, -10.6239) (4.2571, -10.658) (4.2797, -10.692) (4.3027, -10.7258) (4.326, -10.7594) (4.3497, -10.7929) (4.374, -10.826) (4.3989, -10.8589) (4.4244, -10.8914) (4.4505, -10.9236) (4.4772, -10.9556) (4.5042, -10.9873) (4.5316, -11.0189) (4.5593, -11.0502) (4.5874, -11.0814) (4.6159, -11.1123) (4.6447, -11.143) (4.674, -11.1735) (4.7036, -11.2038) (4.7336, -11.2338) (4.7639, -11.2637) (4.7946, -11.2933) (4.8256, -11.3227) (4.8569, -11.352) (4.8885, -11.381) (4.9204, -11.4099) (4.9527, -11.4385) (4.9852, -11.4669) (5.0181, -11.4952) (5.0512, -11.5232) (5.0847, -11.551) (5.1184, -11.5787) (5.1524, -11.6061) (5.1867, -11.6334) (5.2213, -11.6604) (5.2561, -11.6873) (5.2912, -11.7139) (5.3266, -11.7404) (5.3622, -11.7666) (5.3981, -11.7927) (5.4343, -11.8186) (5.4707, -11.8443) (5.5073, -11.8698) (5.5442, -11.8951) (5.5813, -11.9202) (5.6187, -11.9451) (5.6563, -11.9698) (5.6942, -11.9943) (5.7323, -12.0186) (5.7706, -12.0427) (5.8092, -12.0667) (5.848, -12.0904) (5.887, -12.1139) (5.9262, -12.1373) (5.9656, -12.1604) (6.0053, -12.1834) (6.0452, -12.2061) (6.0853, -12.2287) (6.1256, -12.251) (6.1661, -12.2732) (6.2069, -12.2952) (6.2478, -12.3169) (6.2889, -12.3385) (6.3303, -12.3599) (6.3718, -12.3811) (6.4052, -12.3979) (6.4304, -12.4104) (6.4472, -12.4186) (6.4556, -12.4228) knots 0 0 0 0 0 0 0.01428571 0.02857143 0.04285714 0.05714286 0.07142857 0.08571429 0.1 0.11428571 0.12857143 0.14285714 0.15714286 0.17142857 0.18571429 0.2 0.21428571 0.22857143 0.24285714 0.25714286 0.27142857 0.28571429 0.3 0.31428571 0.32857143 0.34285714 0.35714286 0.37142857 0.38571429 0.4 0.41428571 0.42857143 0.44285714 0.45714286 0.47142857 0.48571429 0.5 0.51428571 0.52857143 0.54285714 0.55714286 0.57142857 0.58571429 0.6 0.61428571 0.62857143 0.64285714 0.65714286 0.67142857 0.68571429 0.7 0.71428571 0.72857143 0.74285714 0.75714286 0.77142857 0.78571429 0.8 0.81428571 0.82857143 0.84285714 0.85714286 0.87142857 0.88571429 0.9 0.91428571 0.92857143 0.94285714 0.95714286 0.97142857 0.98571429 1 1 1 1 1 1
  arc A18 (6.4556, -12.4228) -> (7.5307, -11.8021) centre (0, 0) ccw
  spline S9 degree 5 poles (7.5307, -11.8021) (7.5313, -11.7927) (7.5325, -11.774) (7.5342, -11.746) (7.5364, -11.7087) (7.5388, -11.6621) (7.541, -11.6156) (7.5429, -11.5692) (7.5445, -11.5229) (7.5458, -11.4766) (7.5469, -11.4305) (7.5477, -11.3844) (7.5482, -11.3384) (7.5484, -11.2924) (7.5484, -11.2466) (7.5481, -11.2009) (7.5475, -11.1552) (7.5466, -11.1097) (7.5454, -11.0642) (7.544, -11.0189) (7.5423, -10.9736) (7.5403, -10.9285) (7.538, -10.8834) (7.5354, -10.8385) (7.5325, -10.7937) (7.5293, -10.7489) (7.5259, -10.7044) (7.5221, -10.6599) (7.5181, -10.6155) (7.5137, -10.5713) (7.5091, -10.5271) (7.5042, -10.4832) (7.4989, -10.4393) (7.4934, -10.3956) (7.4876, -10.352) (7.4814, -10.3085) (7.475, -10.2652) (7.4682, -10.222) (7.4611, -10.179) (7.4538, -10.1361) (7.4461, -10.0934) (7.438, -10.0508) (7.4297, -10.0084) (7.421, -9.9662) (7.412, -9.9241) (7.4027, -9.8822) (7.393, -9.8404) (7.383, -9.7989) (7.3727, -9.7575) (7.362, -9.7163) (7.351, -9.6753) (7.3396, -9.6345) (7.3278, -9.594) (7.3156, -9.5536) (7.303, -9.5135) (7.2901, -9.4736) (7.2768, -9.4339) (7.2632, -9.3944) (7.2492, -9.3551) (7.2349, -9.3161) (7.22, -9.2774) (7.2046, -9.239) (7.1886, -9.201) (7.172, -9.1634) (7.1549, -9.1261) (7.1374, -9.0891) (7.1196, -9.0523) (7.1016, -9.0157) (7.0831, -8.9794) (7.064, -8.9437) (7.0436, -8.9087) (7.0261, -8.8816) (7.012, -8.862) (7.0022, -8.8491) (6.9972, -8.8428) knots -1 -1 -1 -1 -1 -1 -0.98571429 -0.97142857 -0.95714286 -0.94285714 -0.92857143 -0.91428571 -0.9 -0.88571429 -0.87142857 -0.85714286 -0.84285714 -0.82857143 -0.81428571 -0.8 -0.78571429 -0.77142857 -0.75714286 -0.74285714 -0.72857143 -0.71428571 -0.7 -0.68571429 -0.67142857 -0.65714286 -0.64285714 -0.62857143 -0.61428571 -0.6 -0.58571429 -0.57142857 -0.55714286 -0.54285714 -0.52857143 -0.51428571 -0.5 -0.48571429 -0.47142857 -0.45714286 -0.44285714 -0.42857143 -0.41428571 -0.4 -0.38571429 -0.37142857 -0.35714286 -0.34285714 -0.32857143 -0.31428571 -0.3 -0.28571429 -0.27142857 -0.25714286 -0.24285714 -0.22857143 -0.21428571 -0.2 -0.18571429 -0.17142857 -0.15714286 -0.14285714 -0.12857143 -0.11428571 -0.1 -0.08571429 -0.07142857 -0.05714286 -0.04285714 -0.02857143 -0.01428571 0 0 0 0 0 0
  line L9 (6.9972, -8.8428) -> (6.5164, -8.2343)
  arc A19 (6.609, -6.8926) -> (6.5164, -8.2343) centre (7.3011, -7.6144) ccw
  arc A20 (6.609, -6.8926) -> (6.8926, -6.609) centre (0, 0) ccw
  arc A21 (8.2343, -6.5164) -> (6.8926, -6.609) centre (7.6144, -7.3011) ccw
  line L10 (8.2343, -6.5164) -> (8.8428, -6.9972)
  spline S10 degree 5 poles (8.8428, -6.9972) (8.8491, -7.0022) (8.862, -7.012) (8.8816, -7.0261) (8.9087, -7.0436) (8.9437, -7.064) (8.9794, -7.0831) (9.0157, -7.1016) (9.0523, -7.1196) (9.0891, -7.1374) (9.1261, -7.1549) (9.1634, -7.172) (9.201, -7.1886) (9.239, -7.2046) (9.2774, -7.22) (9.3161, -7.2349) (9.3551, -7.2492) (9.3944, -7.2632) (9.4339, -7.2768) (9.4736, -7.2901) (9.5135, -7.303) (9.5536, -7.3156) (9.594, -7.3278) (9.6345, -7.3396) (9.6753, -7.351) (9.7163, -7.362) (9.7575, -7.3727) (9.7989, -7.383) (9.8404, -7.393) (9.8822, -7.4027) (9.9241, -7.412) (9.9662, -7.421) (10.0084, -7.4297) (10.0508, -7.438) (10.0934, -7.4461) (10.1361, -7.4538) (10.179, -7.4611) (10.222, -7.4682) (10.2652, -7.475) (10.3085, -7.4814) (10.352, -7.4876) (10.3956, -7.4934) (10.4393, -7.4989) (10.4832, -7.5042) (10.5271, -7.5091) (10.5713, -7.5137) (10.6155, -7.5181) (10.6599, -7.5221) (10.7044, -7.5259) (10.7489, -7.5293) (10.7937, -7.5325) (10.8385, -7.5354) (10.8834, -7.538) (10.9285, -7.5403) (10.9736, -7.5423) (11.0189, -7.544) (11.0642, -7.5454) (11.1097, -7.5466) (11.1552, -7.5475) (11.2009, -7.5481) (11.2466, -7.5484) (11.2924, -7.5484) (11.3384, -7.5482) (11.3844, -7.5477) (11.4305, -7.5469) (11.4766, -7.5458) (11.5229, -7.5445) (11.5692, -7.5429) (11.6156, -7.541) (11.6621, -7.5388) (11.7087, -7.5364) (11.746, -7.5342) (11.774, -7.5325) (11.7927, -7.5313) (11.8021, -7.5307) knots 0 0 0 0 0 0 0.01428571 0.02857143 0.04285714 0.05714286 0.07142857 0.08571429 0.1 0.11428571 0.12857143 0.14285714 0.15714286 0.17142857 0.18571429 0.2 0.21428571 0.22857143 0.24285714 0.25714286 0.27142857 0.28571429 0.3 0.31428571 0.32857143 0.34285714 0.35714286 0.37142857 0.38571429 0.4 0.41428571 0.42857143 0.44285714 0.45714286 0.47142857 0.48571429 0.5 0.51428571 0.52857143 0.54285714 0.55714286 0.57142857 0.58571429 0.6 0.61428571 0.62857143 0.64285714 0.65714286 0.67142857 0.68571429 0.7 0.71428571 0.72857143 0.74285714 0.75714286 0.77142857 0.78571429 0.8 0.81428571 0.82857143 0.84285714 0.85714286 0.87142857 0.88571429 0.9 0.91428571 0.92857143 0.94285714 0.95714286 0.97142857 0.98571429 1 1 1 1 1 1
  arc A22 (11.8021, -7.5307) -> (12.4228, -6.4556) centre (0, 0) ccw
  spline S11 degree 5 poles (12.4228, -6.4556) (12.4186, -6.4472) (12.4104, -6.4304) (12.3979, -6.4052) (12.3811, -6.3718) (12.3599, -6.3303) (12.3385, -6.2889) (12.3169, -6.2478) (12.2952, -6.2069) (12.2732, -6.1661) (12.251, -6.1256) (12.2287, -6.0853) (12.2061, -6.0452) (12.1834, -6.0053) (12.1604, -5.9656) (12.1373, -5.9262) (12.1139, -5.887) (12.0904, -5.848) (12.0667, -5.8092) (12.0427, -5.7706) (12.0186, -5.7323) (11.9943, -5.6942) (11.9698, -5.6563) (11.9451, -5.6187) (11.9202, -5.5813) (11.8951, -5.5442) (11.8698, -5.5073) (11.8443, -5.4707) (11.8186, -5.4343) (11.7927, -5.3981) (11.7666, -5.3622) (11.7404, -5.3266) (11.7139, -5.2912) (11.6873, -5.2561) (11.6604, -5.2213) (11.6334, -5.1867) (11.6061, -5.1524) (11.5787, -5.1184) (11.551, -5.0847) (11.5232, -5.0512) (11.4952, -5.0181) (11.4669, -4.9852) (11.4385, -4.9527) (11.4099, -4.9204) (11.381, -4.8885) (11.352, -4.8569) (11.3227, -4.8256) (11.2933, -4.7946) (11.2637, -4.7639) (11.2338, -4.7336) (11.2038, -4.7036) (11.1735, -4.674) (11.143, -4.6447) (11.1123, -4.6159) (11.0814, -4.5874) (11.0502, -4.5593) (11.0189, -4.5316) (10.9873, -4.5042) (10.9556, -4.4772) (10.9236, -4.4505) (10.8914, -4.4244) (10.8589, -4.3989) (10.826, -4.374) (10.7929, -4.3497) (10.7594, -4.326) (10.7258, -4.3027) (10.692, -4.2797) (10.658, -4.2571) (10.6239, -4.2349) (10.5894, -4.2134) (10.5543, -4.1933) (10.5256, -4.1787) (10.5035, -4.1687) (10.4886, -4.1625) (10.4811, -4.1595) knots -1 -1 -1 -1 -1 -1 -0.98571429 -0.97142857 -0.95714286 -0.94285714 -0.92857143 -0.91428571 -0.9 -0.88571429 -0.87142857 -0.85714286 -0.84285714 -0.82857143 -0.81428571 -0.8 -0.78571429 -0.77142857 -0.75714286 -0.74285714 -0.72857143 -0.71428571 -0.7 -0.68571429 -0.67142857 -0.65714286 -0.64285714 -0.62857143 -0.61428571 -0.6 -0.58571429 -0.57142857 -0.55714286 -0.54285714 -0.52857143 -0.51428571 -0.5 -0.48571429 -0.47142857 -0.45714286 -0.44285714 -0.42857143 -0.41428571 -0.4 -0.38571429 -0.37142857 -0.35714286 -0.34285714 -0.32857143 -0.31428571 -0.3 -0.28571429 -0.27142857 -0.25714286 -0.24285714 -0.22857143 -0.21428571 -0.2 -0.18571429 -0.17142857 -0.15714286 -0.14285714 -0.12857143 -0.11428571 -0.1 -0.08571429 -0.07142857 -0.05714286 -0.04285714 -0.02857143 -0.01428571 0 0 0 0 0 0
  line L11 (10.4811, -4.1595) -> (9.7605, -3.8729)
  arc A23 (9.1699, -2.6646) -> (9.7605, -3.8729) centre (10.1302, -2.9437) ccw
  arc A24 (9.1699, -2.6646) -> (9.2737, -2.2773) centre (0, 0) ccw
  arc A25 (10.3893, -1.5263) -> (9.2737, -2.2773) centre (10.2448, -2.5158) ccw
  line L12 (10.3893, -1.5263) -> (11.1567, -1.6383)
  spline S12 degree 5 poles (11.1567, -1.6383) (11.1647, -1.6395) (11.1807, -1.6416) (11.2048, -1.6439) (11.237, -1.6456) (11.2774, -1.6458) (11.318, -1.6445) (11.3587, -1.6423) (11.3994, -1.6396) (11.4401, -1.6366) (11.4809, -1.6333) (11.5218, -1.6295) (11.5626, -1.625) (11.6035, -1.6199) (11.6445, -1.614) (11.6854, -1.6075) (11.7264, -1.6005) (11.7674, -1.5929) (11.8084, -1.585) (11.8494, -1.5766) (11.8905, -1.5678) (11.9315, -1.5587) (11.9725, -1.5491) (12.0135, -1.539) (12.0545, -1.5285) (12.0956, -1.5175) (12.1366, -1.5062) (12.1776, -1.4944) (12.2186, -1.4823) (12.2595, -1.4698) (12.3005, -1.4569) (12.3414, -1.4437) (12.3824, -1.4301) (12.4233, -1.4161) (12.4641, -1.4018) (12.505, -1.3871) (12.5458, -1.372) (12.5866, -1.3566) (12.6274, -1.3409) (12.6681, -1.3248) (12.7088, -1.3084) (12.7495, -1.2917) (12.7902, -1.2746) (12.8308, -1.2572) (12.8713, -1.2395) (12.9119, -1.2215) (12.9523, -1.2031) (12.9928, -1.1844) (13.0332, -1.1654) (13.0735, -1.1461) (13.1138, -1.1265) (13.1541, -1.1066) (13.1943, -1.0863) (13.2345, -1.0658) (13.2746, -1.045) (13.3146, -1.0239) (13.3546, -1.0024) (13.3946, -0.9807) (13.4344, -0.9587) (13.4743, -0.9364) (13.514, -0.9138) (13.5538, -0.8909) (13.5934, -0.8678) (13.633, -0.8443) (13.6725, -0.8206) (13.712, -0.7966) (13.7514, -0.7723) (13.7907, -0.7477) (13.8299, -0.7229) (13.8691, -0.6978) (13.9082, -0.6724) (13.9395, -0.6518) (13.9629, -0.6363) (13.9784, -0.6259) (13.9862, -0.6207) knots 0 0 0 0 0 0 0.01428571 0.02857143 0.04285714 0.05714286 0.07142857 0.08571429 0.1 0.11428571 0.12857143 0.14285714 0.15714286 0.17142857 0.18571429 0.2 0.21428571 0.22857143 0.24285714 0.25714286 0.27142857 0.28571429 0.3 0.31428571 0.32857143 0.34285714 0.35714286 0.37142857 0.38571429 0.4 0.41428571 0.42857143 0.44285714 0.45714286 0.47142857 0.48571429 0.5 0.51428571 0.52857143 0.54285714 0.55714286 0.57142857 0.58571429 0.6 0.61428571 0.62857143 0.64285714 0.65714286 0.67142857 0.68571429 0.7 0.71428571 0.72857143 0.74285714 0.75714286 0.77142857 0.78571429 0.8 0.81428571 0.82857143 0.84285714 0.85714286 0.87142857 0.88571429 0.9 0.91428571 0.92857143 0.94285714 0.95714286 0.97142857 0.98571429 1 1 1 1 1 1
  arc A26 (13.9862, -0.6207) -> (13.9862, 0.6207) centre (0, 0) ccw
  spline S13 degree 5 poles (13.9862, 0.6207) (13.9784, 0.6259) (13.9629, 0.6363) (13.9395, 0.6518) (13.9082, 0.6724) (13.8691, 0.6978) (13.8299, 0.7229) (13.7907, 0.7477) (13.7514, 0.7723) (13.712, 0.7966) (13.6725, 0.8206) (13.633, 0.8443) (13.5934, 0.8678) (13.5538, 0.8909) (13.514, 0.9138) (13.4743, 0.9364) (13.4344, 0.9587) (13.3946, 0.9807) (13.3546, 1.0024) (13.3146, 1.0239) (13.2746, 1.045) (13.2345, 1.0658) (13.1943, 1.0863) (13.1541, 1.1066) (13.1138, 1.1265) (13.0735, 1.1461) (13.0332, 1.1654) (12.9928, 1.1844) (12.9523, 1.2031) (12.9119, 1.2215) (12.8713, 1.2395) (12.8308, 1.2572) (12.7902, 1.2746) (12.7495, 1.2917) (12.7088, 1.3084) (12.6681, 1.3248) (12.6274, 1.3409) (12.5866, 1.3566) (12.5458, 1.372) (12.505, 1.3871) (12.4641, 1.4018) (12.4233, 1.4161) (12.3824, 1.4301) (12.3414, 1.4437) (12.3005, 1.4569) (12.2595, 1.4698) (12.2186, 1.4823) (12.1776, 1.4944) (12.1366, 1.5062) (12.0956, 1.5175) (12.0545, 1.5285) (12.0135, 1.539) (11.9725, 1.5491) (11.9315, 1.5587) (11.8905, 1.5678) (11.8494, 1.5766) (11.8084, 1.585) (11.7674, 1.5929) (11.7264, 1.6005) (11.6854, 1.6075) (11.6445, 1.614) (11.6035, 1.6199) (11.5626, 1.625) (11.5218, 1.6295) (11.4809, 1.6333) (11.4401, 1.6366) (11.3994, 1.6396) (11.3587, 1.6423) (11.318, 1.6445) (11.2774, 1.6458) (11.237, 1.6456) (11.2048, 1.6439) (11.1807, 1.6416) (11.1647, 1.6395) (11.1567, 1.6383) knots -1 -1 -1 -1 -1 -1 -0.98571429 -0.97142857 -0.95714286 -0.94285714 -0.92857143 -0.91428571 -0.9 -0.88571429 -0.87142857 -0.85714286 -0.84285714 -0.82857143 -0.81428571 -0.8 -0.78571429 -0.77142857 -0.75714286 -0.74285714 -0.72857143 -0.71428571 -0.7 -0.68571429 -0.67142857 -0.65714286 -0.64285714 -0.62857143 -0.61428571 -0.6 -0.58571429 -0.57142857 -0.55714286 -0.54285714 -0.52857143 -0.51428571 -0.5 -0.48571429 -0.47142857 -0.45714286 -0.44285714 -0.42857143 -0.41428571 -0.4 -0.38571429 -0.37142857 -0.35714286 -0.34285714 -0.32857143 -0.31428571 -0.3 -0.28571429 -0.27142857 -0.25714286 -0.24285714 -0.22857143 -0.21428571 -0.2 -0.18571429 -0.17142857 -0.15714286 -0.14285714 -0.12857143 -0.11428571 -0.1 -0.08571429 -0.07142857 -0.05714286 -0.04285714 -0.02857143 -0.01428571 0 0 0 0 0 0
  line L13 (11.1567, 1.6383) -> (10.3893, 1.5263)
  arc A27 (9.2737, 2.2773) -> (10.3893, 1.5263) centre (10.2448, 2.5158) ccw
  arc A28 (9.2737, 2.2773) -> (9.1699, 2.6646) centre (0, 0) ccw
  arc A29 (9.7605, 3.8729) -> (9.1699, 2.6646) centre (10.1302, 2.9437) ccw
  line L14 (9.7605, 3.8729) -> (10.4811, 4.1595)
  spline S14 degree 5 poles (10.4811, 4.1595) (10.4886, 4.1625) (10.5035, 4.1687) (10.5256, 4.1787) (10.5543, 4.1933) (10.5894, 4.2134) (10.6239, 4.2349) (10.658, 4.2571) (10.692, 4.2797) (10.7258, 4.3027) (10.7594, 4.326) (10.7929, 4.3497) (10.826, 4.374) (10.8589, 4.3989) (10.8914, 4.4244) (10.9236, 4.4505) (10.9556, 4.4772) (10.9873, 4.5042) (11.0189, 4.5316) (11.0502, 4.5593) (11.0814, 4.5874) (11.1123, 4.6159) (11.143, 4.6447) (11.1735, 4.674) (11.2038, 4.7036) (11.2338, 4.7336) (11.2637, 4.7639) (11.2933, 4.7946) (11.3227, 4.8256) (11.352, 4.8569) (11.381, 4.8885) (11.4099, 4.9204) (11.4385, 4.9527) (11.4669, 4.9852) (11.4952, 5.0181) (11.5232, 5.0512) (11.551, 5.0847) (11.5787, 5.1184) (11.6061, 5.1524) (11.6334, 5.1867) (11.6604, 5.2213) (11.6873, 5.2561) (11.7139, 5.2912) (11.7404, 5.3266) (11.7666, 5.3622) (11.7927, 5.3981) (11.8186, 5.4343) (11.8443, 5.4707) (11.8698, 5.5073) (11.8951, 5.5442) (11.9202, 5.5813) (11.9451, 5.6187) (11.9698, 5.6563) (11.9943, 5.6942) (12.0186, 5.7323) (12.0427, 5.7706) (12.0667, 5.8092) (12.0904, 5.848) (12.1139, 5.887) (12.1373, 5.9262) (12.1604, 5.9656) (12.1834, 6.0053) (12.2061, 6.0452) (12.2287, 6.0853) (12.251, 6.1256) (12.2732, 6.1661) (12.2952, 6.2069) (12.3169, 6.2478) (12.3385, 6.2889) (12.3599, 6.3303) (12.3811, 6.3718) (12.3979, 6.4052) (12.4104, 6.4304) (12.4186, 6.4472) (12.4228, 6.4556) knots 0 0 0 0 0 0 0.01428571 0.02857143 0.04285714 0.05714286 0.07142857 0.08571429 0.1 0.11428571 0.12857143 0.14285714 0.15714286 0.17142857 0.18571429 0.2 0.21428571 0.22857143 0.24285714 0.25714286 0.27142857 0.28571429 0.3 0.31428571 0.32857143 0.34285714 0.35714286 0.37142857 0.38571429 0.4 0.41428571 0.42857143 0.44285714 0.45714286 0.47142857 0.48571429 0.5 0.51428571 0.52857143 0.54285714 0.55714286 0.57142857 0.58571429 0.6 0.61428571 0.62857143 0.64285714 0.65714286 0.67142857 0.68571429 0.7 0.71428571 0.72857143 0.74285714 0.75714286 0.77142857 0.78571429 0.8 0.81428571 0.82857143 0.84285714 0.85714286 0.87142857 0.88571429 0.9 0.91428571 0.92857143 0.94285714 0.95714286 0.97142857 0.98571429 1 1 1 1 1 1
  arc A30 (12.4228, 6.4556) -> (11.8021, 7.5307) centre (0, 0) ccw